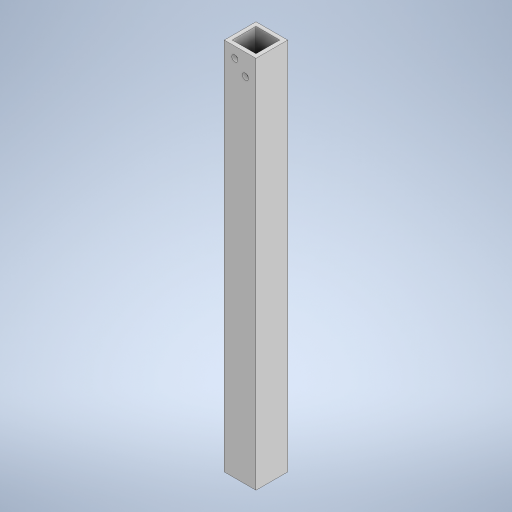
# Autodesk Inventor part: vertical
Saved by Autodesk Inventor 2023 (Build 270158000, 158)
## iProperties
Created: 2023-06-23
Part Number: vertical
Material: Generic
Document SubType Name: Modeling
Designer: incep
Density: 1 g/cm^3
Appearance: Default
Author: incep
Autodesk Inventor part; units mm, degrees
ref_plane "YZ Plane" through (0, 0, 0) normal (1, 0, 0) x (0, 1, 0)
ref_plane "XZ Plane" through (0, 0, 0) normal (0, 1, 0) x (-1, 0, 0)
ref_plane "XY Plane" through (0, 0, 0) normal (0, 0, 1) x (1, 0, 0)
sketch "Sketch1" plane through (0, 0, 0) normal (0, 1, 0) x (-1, 0, 0)
  line L0 (12.7, -12.7) -> (-12.7, -12.7)
  line L1 (-12.7, -12.7) -> (-12.7, 12.7)
  line L2 (-12.7, 12.7) -> (12.7, 12.7)
  line L3 (12.7, 12.7) -> (12.7, -12.7)
  line L4 (9.525, -9.525) -> (-9.525, -9.525)
  line L5 (-9.525, -9.525) -> (-9.525, 9.525)
  line L6 (-9.525, 9.525) -> (9.525, 9.525)
  line L7 (9.525, 9.525) -> (9.525, -9.525)
  point P0 (0, 0)
  point P1 (0, -9.525)
  point P2 (0, -12.7)
  point P3 (-9.525, 0)
  point P4 (-12.7, 0)
  dimension "d0" = 25.4
  dimension "d1" = 3.175
  constraints: 16 end point, 4 midpoint, 4 parallel, 4 perpendicular, 2 horizontal, 2 horizontal alignment, 2 vertical alignment
  measures "d0" distance of L0.start L0.end
  measures "d1" distance between parallel lines of L1 L5
extrude "Extrusion1" add sketch "Sketch1" along normal blind 300
sketch "Sketch2" plane through (-12.7, 0, 12.7) normal (0, 0, 1) x (1, 0, 0)
  line L0 (0, 0) -> (0, 300) construction
  line L1 (0, 300) -> (25.4, 300) construction
  line L2 (25.4, 300) -> (25.4, 274.6) construction
  line L3 (25.4, 274.6) -> (0, 274.6) construction
  line L4 (0, 274.6) -> (0, 300) construction
  line L5 (25.4, 0) -> (25.4, 300) construction
  line L6 (8.4667, 291.5333) -> (16.9333, 291.5333) construction
  line L7 (16.9333, 291.5333) -> (16.9333, 283.0667) construction
  line L8 (16.9333, 283.0667) -> (8.4667, 283.0667) construction
  line L9 (8.4667, 283.0667) -> (8.4667, 291.5333) construction
  circle A0 centre (8.4667, 291.5333) radius 2.4257
  circle A1 centre (16.9333, 283.0667) radius 2.4257
  point P0 (12.7, 0)
  point P1 (12.7, 291.5333)
  point P2 (12.7, 300)
  point P3 (16.9333, 287.3)
  point P4 (25.4, 287.3)
  dimension "d4" = 8.4667
  dimension "d5" = 4.8514
  constraints: 16 end point, 4 midpoint, 4 parallel, 4 perpendicular, 2 centre point, 2 coincident, 2 horizontal, 1 equal radius, 1 horizontal alignment, 1 point on line, 1 vertical alignment
  measures "d4" distance of L6.start L6.end
  measures "d5" diameter of A0
sketch "Sketch3" plane through (-12.7, 0, -12.7) normal (-1, 0, 0) x (0, 0, 1)
  line L0 (0, 0) -> (0, 300) construction
  line L1 (0, 300) -> (25.4, 300) construction
  line L2 (25.4, 300) -> (25.4, 274.6) construction
  line L3 (25.4, 274.6) -> (0, 274.6) construction
  line L4 (0, 274.6) -> (0, 300) construction
  line L5 (8.4667, 291.5333) -> (16.9333, 291.5333) construction
  line L6 (16.9333, 291.5333) -> (16.9333, 283.0667) construction
  line L7 (16.9333, 283.0667) -> (8.4667, 283.0667) construction
  line L8 (8.4667, 283.0667) -> (8.4667, 291.5333) construction
  circle A0 centre (16.9333, 291.5333) radius 2.4257
  circle A1 centre (8.4667, 283.0667) radius 2.4257
  point P0 (12.7, 0)
  point P1 (16.9333, 287.3)
  point P2 (25.4, 287.3)
  point P3 (12.7, 283.0667)
  point P4 (12.7, 274.6)
  dimension "d6" = 25.4
  dimension "d7" = 8.4667
  dimension "d8" = 4.8514
  constraints: 16 end point, 4 midpoint, 4 parallel, 4 perpendicular, 2 centre point, 2 coincident, 2 horizontal, 1 equal radius, 1 horizontal alignment, 1 vertical alignment
  measures "d6" distance of L2.end L3.end
  measures "d7" distance of L6.end L7.end
  measures "d8" diameter of A0
extrude "Extrusion2" cut sketch "Sketch3" against normal blind 3.175
extrude "Extrusion3" cut sketch "Sketch2" against normal blind 3.175
body "Solid1"
